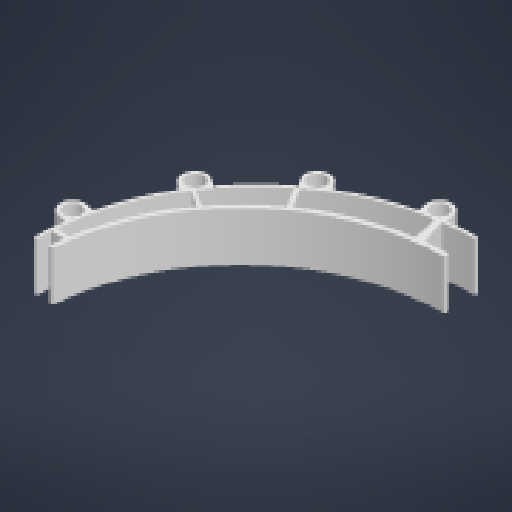
# Autodesk Inventor part: HalfFilterwall2.5
Saved by Autodesk Inventor 2026 (Build 300175050, 175E)
## iProperties
Created: 2026-05-09
Part Number: HalfFilterwall2.5
Material: Generic
Document SubType Name: Modeling
Designer: sniel
Density: 1 g/cm^3
Appearance: Default
Author: sniel
Autodesk Inventor part; units mm, degrees
ref_plane "YZ Plane" through (0, 0, 0) normal (1, 0, 0) x (0, 1, 0)
ref_plane "XZ Plane" through (0, 0, 0) normal (0, 1, 0) x (-1, 0, 0)
ref_plane "XY Plane" through (0, 0, 0) normal (0, 0, 1) x (1, 0, 0)
sketch "Sketch1" plane through (0, 0, 0) normal (0, 1, 0) x (-1, 0, 0)
  line L0 (25.9114, 34.2491) -> (21.2332, 33.3843)
  arc A0 (20.0516, 34.3835) -> (21.2332, 33.3843) centre (21.0514, 34.3676) ccw
  arc A1 (-119.7713, -90.2007) -> (-23.8722, 132.5898) centre (-107.1679, 36.4091) ccw
  arc A2 (26.7278, 35.2912) -> (-23.8722, 132.5898) centre (-107.2761, 27.4091) ccw
  arc A3 (25.9114, 34.2491) -> (26.7278, 35.2912) centre (25.7296, 35.2325) ccw
  line L1 (27.8468, 45.6636) -> (26.3501, 52.6594)
  arc A4 (26.2623, 53.1202) -> (26.3501, 52.6594) centre (31.4582, 53.8718) ccw
  line L2 (26.2623, 53.1202) -> (25.0871, 60.1318)
  arc A5 (25.0871, 60.1318) -> (9.4911, 97.7837) centre (-107.1602, 27.4092) ccw
  line L3 (9.4911, 97.7837) -> (5.3135, 103.6771)
  arc A6 (5.0787, 104.0229) -> (5.3135, 103.6771) centre (9.5358, 106.7971) ccw
  line L4 (5.0787, 104.0229) -> (1.2119, 109.9658)
  arc A7 (1.2119, 109.9658) -> (-24.6037, 135.7814) centre (-107.1602, 27.4092) ccw
  line L5 (-24.6037, 135.7814) -> (-30.7027, 139.7893)
  arc A8 (-30.9761, 139.9752) -> (-30.7027, 139.7893) centre (-27.8881, 144.221) ccw
  line L6 (-30.9761, 139.9752) -> (-36.7857, 144.0605)
  arc A9 (-36.7857, 144.0605) -> (-74.4376, 159.6565) centre (-107.1602, 27.4092) ccw
  line L7 (-74.4376, 159.6565) -> (-81.6968, 160.9683)
  arc A10 (-81.9001, 161.0071) -> (-81.6968, 160.9683) centre (-80.8134, 166.1434) ccw
  line L8 (-81.9001, 161.0071) -> (-88.9058, 162.4162)
  arc A11 (-88.9058, 162.4162) -> (-106.2695, 163.6418) centre (-107.1602, 27.4092) ccw
  arc A12 (-106.2695, 163.6418) -> (-107.2761, 162.6418) centre (-106.2761, 162.6418) ccw
  line L9 (-107.2761, 162.6418) -> (-107.2761, 162.6407)
  arc A13 (-107.2761, 162.6407) -> (-106.284, 161.6407) centre (-106.2761, 162.6407) ccw
  arc A14 (-107.2761, -87.8264) -> (-106.284, 161.6407) centre (-107.2761, 36.9091) ccw
  arc A15 (17.1741, 28.4768) -> (18.1718, 27.4092) centre (18.1718, 28.4092) ccw
  line L10 (18.1718, 27.4092) -> (18.8139, 27.4092)
  arc A16 (18.8139, 27.4092) -> (19.8119, 28.3458) centre (18.8139, 28.4092) ccw
  arc A17 (19.8119, 28.3458) -> (19.9242, 30.3677) centre (-107.1679, 36.4091) ccw
  arc A18 (20.7451, 31.3043) -> (19.9242, 30.3677) centre (20.923, 30.3203) ccw
  line L11 (20.7451, 31.3043) -> (25.727, 32.2051)
  arc A19 (26.9045, 31.2497) -> (25.727, 32.2051) centre (25.9049, 31.2211) ccw
  arc A20 (26.9558, 28.4018) -> (26.9045, 31.2497) centre (-107.2761, 27.4091) ccw
  arc A21 (26.9558, 28.4018) -> (27.9558, 27.4092) centre (27.9558, 28.4092) ccw
  line L12 (27.9558, 27.4092) -> (28.0716, 27.4092)
  arc A22 (28.0716, 27.4092) -> (29.0716, 28.4166) centre (28.0716, 28.4092) ccw
  arc A23 (29.0716, 28.4166) -> (27.8468, 45.6636) centre (-107.1606, 27.4092) ccw
  circle A24 centre (-80.8134, -111.3251) radius 5.25
  circle A25 centre (-27.8881, -89.4028) radius 5.25
  circle A26 centre (31.4582, 0.9465) radius 5.25
  circle A27 centre (9.5358, -51.9789) radius 5.25
  line L13 (-36.9015, -89.2422) -> (-34.2008, -93.4523)
  arc A28 (-34.2008, -93.4523) -> (-21.7991, -85.0238) centre (-27.8881, -89.4028) ccw
  line L14 (-21.7991, -85.0238) -> (-24.7195, -80.9631)
  arc A29 (-24.7195, -80.9631) -> (1.0961, -55.1474) centre (-107.2761, 27.4091) ccw
  line L15 (1.0961, -55.1474) -> (5.1569, -58.0678)
  arc A30 (5.1569, -58.0678) -> (13.5853, -45.6661) centre (9.5358, -51.9789) ccw
  line L16 (13.5853, -45.6661) -> (9.3753, -42.9654)
  arc A31 (9.3753, -42.9654) -> (24.9712, -5.3135) centre (-107.2761, 27.4091) ccw
  line L17 (24.9712, -5.3135) -> (29.8578, -6.3808)
  arc A32 (29.8578, -6.3808) -> (32.6673, 8.3484) centre (31.4582, 0.9465) ccw
  line L18 (32.6673, 8.3484) -> (27.7309, 9.1547)
  arc A33 (27.7309, 9.1547) -> (28.9594, 27.4091) centre (-107.2761, 27.4091) ccw
  line L19 (28.9594, 27.4091) -> (26.9594, 27.4091)
  arc A34 (-107.2761, -106.8264) -> (26.9594, 27.4091) centre (-107.2761, 27.4091) ccw
  line L20 (-107.2761, -106.8264) -> (-107.2761, -108.8264)
  arc A35 (-107.2761, -108.8264) -> (-89.0217, -107.5979) centre (-107.2761, 27.4091) ccw
  line L21 (-89.0217, -107.5979) -> (-88.2153, -112.5343)
  arc A36 (-88.2153, -112.5343) -> (-73.4861, -109.7248) centre (-80.8134, -111.3251) ccw
  line L22 (-73.4861, -109.7248) -> (-74.5534, -104.8382)
  arc A37 (-74.5534, -104.8382) -> (-36.9015, -89.2422) centre (-107.2761, 27.4091) ccw
  arc A38 (-242.2831, 45.6635) -> (-241.3846, 3.4293) centre (-107.2761, 27.4091) ccw
  arc A39 (-240.7954, 0.3407) -> (-241.3846, 3.4293) centre (-246.0104, 0.9465) ccw
  arc A40 (-240.7954, 0.3407) -> (-220.8288, -47.863) centre (-107.2761, 27.4091) ccw
  arc A41 (-219.0614, -50.4636) -> (-220.8288, -47.863) centre (-224.088, -51.9789) ccw
  arc A42 (-219.0614, -50.4636) -> (-185.1488, -84.3762) centre (-107.2761, 27.4091) ccw
  arc A43 (-182.5482, -86.1436) -> (-185.1488, -84.3762) centre (-186.6641, -89.4028) ccw
  arc A44 (-182.5482, -86.1436) -> (-134.3445, -106.1102) centre (-107.2761, 27.4091) ccw
  arc A45 (-131.2559, -106.6994) -> (-134.3445, -106.1102) centre (-133.7387, -111.3251) ccw
  arc A46 (-131.2559, -106.6994) -> (-107.2761, -108.8264) centre (-107.2761, 27.4091) ccw
  line L23 (-107.2761, -108.8264) -> (-107.2761, -106.8264)
  arc A47 (-121.4579, -106.0751) -> (-107.2761, -106.8264) centre (-107.2761, 27.4091) ccw
  arc A48 (-123.445, -105.849) -> (-121.4579, -106.0751) centre (-107.2761, 27.4091) ccw
  arc A49 (-157.8226, -96.9461) -> (-123.445, -105.849) centre (-107.2761, 27.4091) ccw
  arc A50 (-159.6697, -96.1792) -> (-157.8226, -96.9461) centre (-107.2761, 27.4091) ccw
  arc A51 (-206.2357, -63.2891) -> (-159.6697, -96.1792) centre (-107.2761, 27.4091) ccw
  arc A52 (-207.576, -61.8047) -> (-206.2357, -63.2891) centre (-107.2761, 27.4091) ccw
  arc A53 (-239.25, 2.8723) -> (-207.576, -61.8047) centre (-107.2761, 27.4091) ccw
  line L24 (-239.25, 2.8723) -> (-207.9299, 9.4178)
  arc A54 (-207.6519, 3.0359) -> (-207.9299, 9.4178) centre (-239.6009, 4.8412) ccw
  arc A55 (-207.6519, 3.0359) -> (-188.343, -44.3307) centre (-112.1005, 14.3682) ccw
  line L25 (-188.343, -44.3307) -> (-207.576, -61.8047)
  line L26 (-207.576, -61.8047) -> (-206.2357, -63.2891)
  line L27 (-206.2357, -63.2891) -> (-186.0453, -47.223)
  arc A56 (-186.0453, -47.223) -> (-151.3874, -76.2303) centre (-92.213, 29.6796) ccw
  line L28 (-151.3874, -76.2303) -> (-159.6697, -96.1792)
  line L29 (-159.6697, -96.1792) -> (-157.8226, -96.9461)
  line L30 (-157.8226, -96.9461) -> (-149.6232, -77.1969)
  arc A57 (-149.6232, -77.1969) -> (-121.5364, -88.0432) centre (-92.213, 29.6796) ccw
  line L31 (-121.5364, -88.0432) -> (-123.445, -105.849)
  line L32 (-123.445, -105.849) -> (-121.4579, -106.0751)
  line L33 (-121.4579, -106.0751) -> (-119.5917, -88.5106)
  arc A58 (-119.5917, -88.5106) -> (-107.2761, -90.7015) centre (-92.213, 29.6796) ccw
  line L34 (-107.2761, -90.7015) -> (-107.2761, -87.6913)
  arc A59 (-186.1224, -42.3132) -> (-107.2761, -87.6913) centre (-90.977, 31.8176) ccw
  arc A60 (-206.3171, 11.7828) -> (-186.1224, -42.3132) centre (-103.2136, 19.455) ccw
  arc A61 (-206.3171, 11.7828) -> (-242.2831, 45.6635) centre (-244.8864, 6.8698) ccw
  line L35 (-107.2761, -87.8264) -> (-107.2761, -106.8264)
  line L36 (26.9594, 27.4091) -> (17.0972, 27.4091)
  line L37 (26.6723, 18.6343) -> (18.8722, 19.0084)
  line L38 (18.8722, 19.0084) -> (18.4269, 16.0417)
  line L39 (18.4269, 16.0417) -> (26.444, 15.6571)
  line L40 (16.4781, -24.5917) -> (6.8905, -19.9785)
  line L41 (6.8905, -19.9785) -> (5.5294, -22.652)
  line L42 (5.5294, -22.652) -> (15.2844, -27.3458)
  line L43 (-7.6811, -62.591) -> (-16.7091, -53.0677)
  line L44 (-16.7091, -53.0677) -> (-18.8438, -55.1755)
  line L45 (-18.8438, -55.1755) -> (-9.7214, -64.7985)
  line L46 (-101.5313, -90.7015) -> (-101.5313, -106.7034)
  line L47 (-101.5313, -106.7034) -> (-98.5357, -106.5415)
  line L48 (-98.5357, -106.5415) -> (-98.5357, -90.5333)
  point P0 (0, 0)
  point P1 (19.749, 27.4091)
  point P2 (-107.2761, -90.7015)
  point P3 (-107.2761, -90.8264)
  point P4 (-107.2761, -90.7015)
  dimension "d0" = 3
  dimension "d1" = 3
  dimension "d2" = 3
  dimension "d3" = 3
  constraints: 114 point on circle, 98 end point, 60 centre point, 4 parallel, 2 point on line, 2 vertical, 1 horizontal, 26 other
  measures "d0" distance of L37.end L38.end
  measures "d1" distance of L40.end L41.end
  measures "d2" distance of L43.end L44.end
  measures "d3" distance of L46.end L47.end
extrude "Extrusion1" add sketch "Sketch1" along normal blind 30 contours A1 L35 L34 A14 L36 L10 L38 L44 | A34 L19 L12 A33 L18 A32 L17 A31 L16 A30 L15 A29 L14 A28 L13 A37 L22 A36 L21 A35 L20 | L44 A1 | L38 A1 | A1 L37 A34 L39
sketch "Sketch2" plane through (0, 30, 0) normal (0, 1, 0) x (1, 0, 0)
  arc A0 (-26.6723, -18.6343) -> (-26.9594, -27.4091) centre (107.2761, -27.4091) ccw projected
  line L0 (-26.6723, -18.6343) -> (-18.8722, -19.0084) projected
  arc A1 (-18.8722, -19.0084) -> (-19.749, -27.4091) centre (107.1679, -36.4091) ccw projected
  line L1 (-19.749, -27.4091) -> (-17.0972, -27.4091) projected
  arc A2 (107.2761, 87.8264) -> (-17.0972, -27.4091) centre (107.2761, -36.9091) ccw projected
  line L2 (107.2761, 87.8264) -> (107.2761, 90.8264) projected
  arc A3 (107.2761, 90.8264) -> (-18.4269, -16.0417) centre (107.1679, -36.4091) ccw projected
  line L3 (-18.4269, -16.0417) -> (-26.444, -15.6571) projected
  arc A4 (107.2761, 106.8264) -> (-26.444, -15.6571) centre (107.2761, -27.4091) ccw projected
  line L4 (107.2761, 106.8264) -> (107.2761, 108.8264) projected
  arc A5 (107.2761, 108.8264) -> (89.0217, 107.5979) centre (107.2761, -27.4091) ccw projected
  line L5 (89.0217, 107.5979) -> (88.2153, 112.5343) projected
  arc A6 (88.2153, 112.5343) -> (73.4861, 109.7248) centre (80.8134, 111.3251) ccw projected
  line L6 (73.4861, 109.7248) -> (74.5534, 104.8382) projected
  arc A7 (74.5534, 104.8382) -> (36.9015, 89.2422) centre (107.2761, -27.4091) ccw projected
  line L7 (36.9015, 89.2422) -> (34.2008, 93.4523) projected
  arc A8 (34.2008, 93.4523) -> (21.7991, 85.0238) centre (27.8881, 89.4028) ccw projected
  line L8 (21.7991, 85.0238) -> (24.7195, 80.9631) projected
  arc A9 (24.7195, 80.9631) -> (-1.0961, 55.1474) centre (107.2761, -27.4091) ccw projected
  line L9 (-1.0961, 55.1474) -> (-5.1569, 58.0678) projected
  arc A10 (-5.1569, 58.0678) -> (-13.5853, 45.6661) centre (-9.5358, 51.9789) ccw projected
  line L10 (-13.5853, 45.6661) -> (-9.3753, 42.9654) projected
  arc A11 (-9.3753, 42.9654) -> (-24.9712, 5.3135) centre (107.2761, -27.4091) ccw projected
  line L11 (-24.9712, 5.3135) -> (-29.8578, 6.3808) projected
  arc A12 (-29.8578, 6.3808) -> (-32.6673, -8.3484) centre (-31.4582, -0.9465) ccw projected
  line L12 (-32.6673, -8.3484) -> (-27.7309, -9.1547) projected
  arc A13 (-27.7309, -9.1547) -> (-28.9594, -27.4091) centre (107.2761, -27.4091) ccw projected
  line L13 (-28.9594, -27.4091) -> (-26.9594, -27.4091) projected
  circle A14 centre (-9.5358, 51.9789) radius 5.25 projected
  circle A15 centre (-31.4582, -0.9465) radius 5.25 projected
  circle A16 centre (27.8881, 89.4028) radius 5.25 projected
  circle A17 centre (80.8134, 111.3251) radius 5.25 projected
  line L14 (84.2581, 104.8382) -> (88.1874, 89.4028)
  line L15 (88.1786, 105.461) -> (92.9637, 90.0311)
  line L16 (24.7195, 78.4379) -> (32.3668, 66.5165)
  line L17 (26.7865, 80.0181) -> (34.4823, 68.0212)
  line L18 (-5.3258, 45.6661) -> (4.8086, 39.1651)
  line L19 (-4.23, 47.3275) -> (6.0064, 40.7611)
  point P0 (0, 0)
  constraints: 12 end point, 12 point on circle, 2 parallel
extrude "Extrusion2" add sketch "Sketch2" against normal blind 30 contours A3 L14 A4 L15 | A3 L16 A4 L17 | A3 L18 A4 L19
fillet "Fillet1" radius 1 8 edges at (-28.9594, 15, 27.4091) (-26.9594, 15, 27.4091) (-17.0972, 15, 27.4091) (-19.749, 15, 27.4091) (107.2761, 15, -87.8264) (107.2761, 15, -90.8264) (107.2761, 15, -106.8264) (107.2761, 15, -108.8264)
body "Solid1"
